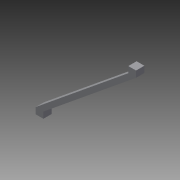
# Autodesk Inventor part: 1Pieceshortsupport_v1
Saved by Autodesk Inventor 2013 (Build 170138000, 138)
## iProperties
Created: 2013-01-19
Part Number: 1Pieceshortsupport_v1
Material: Generic
Document SubType Name: Modeling
Designer: motoennies
Density: 1 g/cm^3
Author: motoennies
Autodesk Inventor part; units mm, degrees
ref_plane "YZ Plane" through (0, 0, 0) normal (1, 0, 0) x (0, 1, 0)
ref_plane "XZ Plane" through (0, 0, 0) normal (0, 1, 0) x (-1, 0, 0)
ref_plane "XY Plane" through (0, 0, 0) normal (0, 0, 1) x (1, 0, 0)
sketch "Sketch1" plane through (0, 0, 0) normal (0, 0, 1) x (1, 0, 0)
  line L0 (0, 0) -> (9.525, 0)
  line L1 (9.525, 0) -> (9.525, 7.62)
  line L2 (0, 0) -> (0, 7.62)
  line L3 (113.3602, 100.1522) -> (113.3602, 107.7722)
  line L4 (113.3602, 107.7722) -> (122.8852, 107.7722)
  line L5 (122.8852, 107.7722) -> (122.8852, 100.1522)
  line L6 (9.525, 7.62) -> (122.8852, 100.1522)
  line L7 (113.3602, 100.1522) -> (0, 7.62)
  dimension "d0" = 9.525
  dimension "d1" = 7.62
  dimension "d2" = 7.62
  dimension "d3" = 9.525
  dimension "d4" = 103.8352
  dimension "d5" = 92.5322
  dimension "d6" = 7.62
  constraints: 16 end point, 4 parallel, 2 perpendicular, 1 horizontal
  measures "d0" distance of L0.start L0.end
  measures "d1" distance of L0.end L1.end
  measures "d2" distance of L3.start L3.end
  measures "d3" distance of L3.end L4.end
  measures "d4" distance between parallel lines of L3 L1
  measures "d5" vertical distance of L2.end L3.start
  measures "d6" distance of L4.end L5.end
extrude "Extrusion1" add sketch "Sketch1" along normal blind 10.16
body "Solid1"
